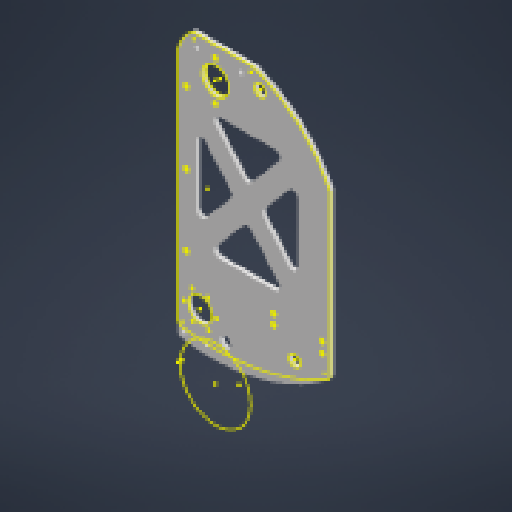
# Autodesk Inventor part: стенка пуляло ответная
Saved by Autodesk Inventor 2026.2 (Build 302298000, 298)
## iProperties
Created: 2025-11-22
Part Number: стенка пуляло ответная
Material: Типовые
Document SubType Name: Modeling
Designer: Phantom
Density: 1 g/cm^3
Appearance: По умолчанию
Author: Phantom
Autodesk Inventor part; units mm, degrees
ref_plane "YZ Plane" through (0, 0, 0) normal (1, 0, 0) x (0, 1, 0)
ref_plane "XZ Plane" through (0, 0, 0) normal (0, 1, 0) x (-1, 0, 0)
ref_plane "XY Plane" through (0, 0, 0) normal (0, 0, 1) x (1, 0, 0)
sketch "Эскиз1" plane through (0, 0, 0) normal (0, 0, 1) x (1, 0, 0)
  line L0 (0, 0) -> (150, 0)
  line L1 (150, 0) -> (150, 380)
  line L2 (150, 380) -> (0, 380)
  line L3 (0, 380) -> (0, 0)
  dimension "d2" = 150
  dimension "d3" = 380
  constraints: 8 end point, 2 parallel, 1 horizontal, 1 perpendicular
  measures "d2" distance of L1.end L2.end
  measures "d3" distance of L2.end L0.start
extrude "Выдавливание1" add sketch "Эскиз1" along normal blind 4
sketch "Эскиз3" plane through (0, 0, 0) normal (0, 0, -1) x (-1, 0, 0)
  circle A0 centre (-37, 259.345) radius 3.25
  line L0 (-150, 380) -> (0, 380) projected
  line L1 (0, 380) -> (0, 0) projected
  circle A1 centre (-37, 259.345) radius 203.5
  line L2 (-162.8639, 128.9118) -> (-165.6991, 126.0733) projected
  arc A2 (-165.6991, 126.0733) -> (-166.6166, 122.0185) centre (-139.5582, 118.0273) ccw projected
  arc A3 (-166.6166, 122.0185) -> (-165.4337, 121.2858) centre (-47.0897, 313.6766) ccw projected
  arc A4 (-165.4337, 121.2858) -> (-162.2121, 123.9136) centre (-181.0608, 143.7331) ccw projected
  arc A5 (-162.2121, 123.9136) -> (-161.041, 123.208) centre (-47.0897, 313.6766) ccw projected
  arc A6 (-161.041, 123.208) -> (-161.8583, 119.1318) centre (-134.7098, 115.8085) ccw projected
  arc A7 (-161.8583, 119.1318) -> (-160.6577, 118.4286) centre (-47.0897, 313.6766) ccw projected
  arc A8 (-160.6577, 118.4286) -> (-157.5019, 121.1349) centre (-176.8332, 140.484) ccw projected
  arc A9 (-157.5019, 121.1349) -> (-156.3138, 120.4584) centre (-47.0897, 313.6766) ccw projected
  arc A10 (-156.3138, 120.4584) -> (-157.0304, 116.3633) centre (-129.8082, 113.7098) ccw projected
  arc A11 (-157.0304, 116.3633) -> (-155.8129, 115.6898) centre (-47.0897, 313.6766) ccw projected
  arc A12 (-155.8129, 115.6898) -> (-152.7247, 118.473) centre (-172.5268, 137.34) ccw projected
  arc A13 (-152.7247, 118.473) -> (-151.5202, 117.826) centre (-47.0897, 313.6766) ccw projected
  arc A14 (-151.5202, 117.826) -> (-152.1357, 113.7145) centre (-124.8564, 111.7326) ccw projected
  arc A15 (-152.1357, 113.7145) -> (-150.902, 113.0712) centre (-47.0897, 313.6766) ccw projected
  arc A16 (-150.902, 113.0712) -> (-147.8833, 115.9297) centre (-168.1442, 134.3031) ccw projected
  arc A17 (-147.8833, 115.9297) -> (-146.6632, 115.3126) centre (-47.0897, 313.6766) ccw projected
  arc A18 (-146.6632, 115.3126) -> (-147.1773, 111.1871) centre (-119.8574, 109.8779) ccw projected
  arc A19 (-147.1773, 111.1871) -> (-145.928, 110.5745) centre (-47.0897, 313.6766) ccw projected
  arc A20 (-145.928, 110.5745) -> (-142.9807, 113.5064) centre (-163.6882, 131.375) ccw projected
  arc A21 (-142.9807, 113.5064) -> (-141.7458, 112.9195) centre (-47.0897, 313.6766) ccw projected
  arc A22 (-141.7458, 112.9195) -> (-142.1581, 108.7827) centre (-114.8143, 108.1469) ccw projected
  arc A23 (-142.1581, 108.7827) -> (-140.8941, 108.201) centre (-47.0897, 313.6766) ccw projected
  arc A24 (-140.8941, 108.201) -> (-138.0199, 111.2047) centre (-159.1613, 128.5577) ccw projected
  arc A25 (-138.0199, 111.2047) -> (-136.771, 110.6484) centre (-47.0897, 313.6766) ccw projected
  arc A26 (-136.771, 110.6484) -> (-137.0811, 106.5027) centre (-109.73, 106.5408) ccw projected
  arc A27 (-137.0811, 106.5027) -> (-135.8033, 105.9522) centre (-47.0897, 313.6766) ccw projected
  arc A28 (-135.8033, 105.9522) -> (-133.0039, 109.0259) centre (-154.5665, 125.8527) ccw projected
  arc A29 (-133.0039, 109.0259) -> (-131.7416, 108.5005) centre (-47.0897, 313.6766) ccw projected
  arc A30 (-131.7416, 108.5005) -> (-131.9496, 104.3484) centre (-104.6077, 105.0603) ccw projected
  arc A31 (-131.9496, 104.3484) -> (-130.6585, 103.8296) centre (-47.0897, 313.6766) ccw projected
  arc A32 (-130.6585, 103.8296) -> (-127.9358, 106.9713) centre (-149.9063, 123.2618) ccw projected
  arc A33 (-127.9358, 106.9713) -> (-126.6609, 106.4772) centre (-47.0897, 313.6766) ccw projected
  arc A34 (-126.6609, 106.4772) -> (-126.7665, 102.3212) centre (-99.4504, 103.7066) ccw projected
  arc A35 (-126.7665, 102.3212) -> (-125.4631, 101.8344) centre (-47.0897, 313.6766) ccw projected
  arc A36 (-125.4631, 101.8344) -> (-122.8185, 105.0422) centre (-145.1838, 120.7864) ccw projected
  arc A37 (-122.8185, 105.0422) -> (-121.5319, 104.5796) centre (-47.0897, 313.6766) ccw projected
  arc A38 (-121.5319, 104.5796) -> (-121.5351, 100.4223) centre (-94.2614, 102.4803) ccw projected
  arc A39 (-121.5351, 100.4223) -> (-120.22, 99.9678) centre (-47.0897, 313.6766) ccw projected
  arc A40 (-120.22, 99.9678) -> (-117.6553, 103.2397) centre (-140.4017, 118.4282) ccw projected
  arc A41 (-117.6553, 103.2397) -> (-116.3577, 102.8091) centre (-47.0897, 313.6766) ccw projected
  arc A42 (-116.3577, 102.8091) -> (-116.2584, 98.6529) centre (-89.0438, 101.3822) ccw projected
  arc A43 (-116.2584, 98.6529) -> (-114.9326, 98.2309) centre (-47.0897, 313.6766) ccw projected
  arc A44 (-114.9326, 98.2309) -> (-112.4493, 101.5651) centre (-135.5629, 116.1885) ccw projected
  arc A45 (-112.4493, 101.5651) -> (-111.1414, 101.1665) centre (-47.0897, 313.6766) ccw projected
  arc A46 (-111.1414, 101.1665) -> (-110.9398, 97.014) centre (-83.8006, 100.413) ccw projected
  arc A47 (-110.9398, 97.014) -> (-109.604, 96.6248) centre (-47.0897, 313.6766) ccw projected
  arc A48 (-109.604, 96.6248) -> (-107.2035, 100.0192) centre (-130.6705, 114.0687) ccw projected
  arc A49 (-107.2035, 100.0192) -> (-105.8863, 99.6529) centre (-47.0897, 313.6766) ccw projected
  arc A50 (-105.8863, 99.6529) -> (-105.5824, 95.5067) centre (-78.5352, 99.5733) ccw projected
  arc A51 (-105.5824, 95.5067) -> (-104.2374, 95.1505) centre (-47.0897, 313.6766) ccw projected
  arc A52 (-104.2374, 95.1505) -> (-101.9213, 98.603) centre (-125.7273, 112.0701) ccw projected
  arc A53 (-101.9213, 98.603) -> (-100.5954, 98.2693) centre (-47.0897, 313.6766) ccw projected
  arc A54 (-100.5954, 98.2693) -> (-100.1895, 94.1318) centre (-73.2507, 98.8635) ccw projected
  arc A55 (-100.1895, 94.1318) -> (-98.8361, 93.8089) centre (-47.0897, 313.6766) ccw projected
  arc A56 (-98.8361, 93.8089) -> (-96.6058, 97.3173) centre (-120.7363, 110.1938) ccw projected
  arc A57 (-96.6058, 97.3173) -> (-95.2721, 97.0164) centre (-47.0897, 313.6766) ccw projected
  arc A58 (-95.2721, 97.0164) -> (-94.7644, 92.8902) centre (-67.9503, 98.2842) ccw projected
  arc A59 (-94.7644, 92.8902) -> (-93.4034, 92.6007) centre (-47.0897, 313.6766) ccw projected
  arc A60 (-93.4034, 92.6007) -> (-91.2602, 96.1631) centre (-115.7007, 108.4411) ccw projected
  arc A61 (-91.2602, 96.1631) -> (-89.9195, 95.8951) centre (-47.0897, 313.6766) ccw projected
  arc A62 (-89.9195, 95.8951) -> (-89.3103, 91.7826) centre (-62.6373, 97.8356) ccw projected
  arc A63 (-89.3103, 91.7826) -> (-88.2236, 91.5786) centre (-47.0897, 313.6766) ccw projected
  line L3 (-88.2236, 91.5786) -> (-86.0083, 96.7219) projected
  line L4 (-86.0083, 96.7219) -> (-85.0766, 98.9705) projected
  arc A64 (-162.8639, 128.9118) -> (-85.0766, 98.9705) centre (-47.0897, 313.6766) ccw projected
  circle A65 centre (-47.0897, 313.6766) radius 225.875
  line L5 (-145.5079, 77.1409) -> (-145.5079, 75.5909) projected
  arc A66 (-145.5079, 75.5909) -> (-144.0079, 74.0909) centre (-144.0079, 75.5909) ccw projected
  line L6 (-144.0079, 74.0909) -> (-92.7079, 74.0909) projected
  arc A67 (-92.7079, 74.0909) -> (-91.2079, 75.5909) centre (-92.7079, 75.5909) ccw projected
  line L7 (-91.2079, 75.5909) -> (-91.2079, 77.1409) projected
  line L8 (-91.2079, 77.1409) -> (-93.3271, 77.1409) projected
  arc A68 (-93.3271, 81.1409) -> (-93.3271, 77.1409) centre (-94.3579, 79.1409) ccw projected
  line L9 (-93.3271, 81.1409) -> (-91.2079, 81.1409) projected
  line L10 (-91.2079, 81.1409) -> (-91.2079, 87.0409) projected
  line L11 (-91.2079, 87.0409) -> (-93.3271, 87.0409) projected
  arc A69 (-93.3271, 91.0409) -> (-93.3271, 87.0409) centre (-94.3579, 89.0409) ccw projected
  line L12 (-93.3271, 91.0409) -> (-91.2079, 91.0409) projected
  line L13 (-91.2079, 91.0409) -> (-91.2079, 92.5909) projected
  arc A70 (-91.2079, 92.5909) -> (-92.7079, 94.0909) centre (-92.7079, 92.5909) ccw projected
  line L14 (-92.7079, 94.0909) -> (-144.0079, 94.0909) projected
  arc A71 (-144.0079, 94.0909) -> (-145.5079, 92.5909) centre (-144.0079, 92.5909) ccw projected
  line L15 (-145.5079, 92.5909) -> (-145.5079, 91.0409) projected
  line L16 (-145.5079, 91.0409) -> (-143.3887, 91.0409) projected
  arc A72 (-143.3887, 87.0409) -> (-143.3887, 91.0409) centre (-142.3579, 89.0409) ccw projected
  line L17 (-143.3887, 87.0409) -> (-145.5079, 87.0409) projected
  line L18 (-145.5079, 87.0409) -> (-145.5079, 81.1409) projected
  line L19 (-145.5079, 81.1409) -> (-143.3887, 81.1409) projected
  arc A73 (-143.3887, 77.1409) -> (-143.3887, 81.1409) centre (-142.3579, 79.1409) ccw projected
  line L20 (-143.3887, 77.1409) -> (-145.5079, 77.1409) projected
  line L21 (-99.5079, 94.0709) -> (-137.8079, 94.0709) projected
  arc A74 (-98.5279, 93.0909) -> (-99.5079, 94.0709) centre (-99.5079, 93.0909) ccw projected
  line L22 (-98.5279, 75.0909) -> (-98.5279, 93.0909) projected
  arc A75 (-99.5079, 74.1109) -> (-98.5279, 75.0909) centre (-99.5079, 75.0909) ccw projected
  line L23 (-137.8079, 74.1109) -> (-99.5079, 74.1109) projected
  arc A76 (-138.7879, 75.0909) -> (-137.8079, 74.1109) centre (-137.8079, 75.0909) ccw projected
  line L24 (-138.7879, 93.0909) -> (-138.7879, 75.0909) projected
  arc A77 (-137.8079, 94.0709) -> (-138.7879, 93.0909) centre (-137.8079, 93.0909) ccw projected
  circle A78 centre (-142.3579, 79.1409) radius 2.25
  circle A79 centre (-142.3579, 89.0409) radius 2.25
  circle A80 centre (-94.3579, 79.1409) radius 2.25
  circle A81 centre (-94.3579, 89.0409) radius 2.25
  circle A82 centre (-37, 259.345) radius 13.25
  line L25 (-37, 259.345) -> (-37, 239.745)
  line L26 (-37, 239.745) -> (-37, 278.945)
  circle A83 centre (-37, 239.745) radius 2.1
  circle A84 centre (-37, 278.945) radius 2.1
  circle A85 centre (-22.0897, 66.1445) radius 19.3809
  line L27 (-22.0897, 66.1445) -> (-22.0897, 37.9965)
  circle A86 centre (-22.0897, 56.392) radius 12
  circle A87 centre (-13.8706, 70.1196) radius 1.6
  circle A88 centre (-6.0917, 56.1378) radius 1.6
  circle A89 centre (-14.3108, 42.4102) radius 1.6
  circle A90 centre (-30.3088, 42.6644) radius 1.6
  circle A91 centre (-38.0877, 56.6461) radius 1.6
  circle A92 centre (-29.8686, 70.3737) radius 1.6
  point P0 (-22.0897, 56.392)
  point P1 (-22.0897, 56.392)
  dimension "d7" = 407
  dimension "d4" = 6.5
  dimension "d5" = 120.655
  dimension "d6" = 37
  dimension "d10" = 26.5
  dimension "d11" = 19.6
  dimension "d12" = 39.2
  dimension "d13" = 4.2
  dimension "d14" = 4.2
  constraints: 16 centre point, 9 coincident, 6 end point, 4 concentric, 2 point on line, 2 vertical, 8 other
  measures "d4" diameter of A0
  measures "d5" distance from line of L0 A0.centre
  measures "d6" distance from line of L1 A0.centre
  measures "d10" diameter of A82
  measures "d11" distance of L25.start L25.end
  measures "d12" distance of L25.end L26.end
  measures "d13" diameter of A83
  measures "d14" diameter of A84
extrude "Выдавливание2" cut sketch "Эскиз3" against normal blind 10 contours A0 L25 L26 | L26 L25 A0 | A86 A85 L27 A1 | A1 A86 | A88 A85 | A85 A88 | L27 A85 A86 A1 | A91 A1 A85 | A85 A1 A91 | L27 A86 A85 | A85 A86 L27 | A91 A85 A1 | A85 A91 A1 | A81 A69 | A79 A72 | A73 A78 | A80 A68 | A87 | A89 | A90 | A92
sketch "Эскиз4" plane through (0, 0, 0) normal (0, 0, -1) x (-1, 0, 0)
  circle A0 centre (-37, 259.345) radius 13.25 projected
  circle A1 centre (-37, 278.945) radius 2.1 projected
  circle A2 centre (-37, 239.745) radius 2.1 projected
  point P0 (0, 0)
extrude "Выдавливание3" cut sketch "Эскиз3" against normal blind 10 contours A0 L25 L26 | A0 L26 A82 L25 | L26 L25 A0 | A0 L25 A82 L26 | A83 | A84
sketch "Эскиз5" plane through (150, 0, 0) normal (1, 0, 0) x (0, 0, -1)
  line L0 (-4, 380) -> (-4, 0) projected
  line L1 (-4, 30) -> (0, 30)
  line L2 (0, 0) -> (-4, 0) projected
  line L3 (-4, 290) -> (0, 290)
  line L4 (0, 0) -> (0, 380) projected
  line L5 (0, 380) -> (-4, 380) projected
  dimension "d17" = 30
  dimension "d18" = 90
  constraints: 4 end point, 3 point on line, 1 horizontal, 1 perpendicular
  measures "d17" distance between parallel lines of L2 L1
  measures "d18" distance between parallel lines of L3 L5
extrude "Выдавливание4" cut sketch "Эскиз5" against normal through all contours L5 L4 L3 L0 | L1 L4 L2 L0
sketch "Эскиз6" plane through (0, 0, 0) normal (0, 0, -1) x (-1, 0, 0)
  circle A0 centre (-37, 259.345) radius 13.25 projected
  circle A1 centre (-37, 259.345) radius 229.345
  line L0 (0, 30) -> (-150, 30) projected
  circle A2 centre (-37, 259.345) radius 37.9855
  line L1 (-150, 30) -> (-150, 290) projected
  arc A3 (-40.2154, 297.1942) -> (-150, 221.3595) centre (-28.8449, 163.3493) ccw
  circle A4 centre (-142.3579, 89.0409) radius 2.25 projected
  circle A5 centre (-94.3579, 79.1409) radius 2.25 projected
  circle A6 centre (-142.3579, 79.1409) radius 2.25 projected
  circle A7 centre (-94.3579, 89.0409) radius 2.25 projected
  circle A8 centre (-37, 259.345) radius 13.25 projected
  circle A9 centre (-37, 278.945) radius 2.1 projected
  circle A10 centre (-37, 239.745) radius 2.1 projected
  line L2 (0, 290) -> (-150, 290) projected
  line L3 (-150, 30) -> (-150, 290) projected
  line L4 (-150, 30) -> (0, 30) projected
  line L5 (0, 290) -> (0, 30) projected
  point P0 (0, 0)
  point P1 (0, 267.9415)
  point P2 (-14.5685, 290)
  point P3 (-73.6036, 290)
  point P4 (0, 33.0043)
  point P5 (-37, 30)
  point P6 (-150, 59.7701)
  constraints: 2 centre point, 2 coincident, 2 point on circle, 1 point on line, 1 tangent, 4 other
extrude "Выдавливание5" cut sketch "Эскиз6" against normal blind 10 contours A1 L0 L1 | L5 L0 A1 | L1 L2 A3 | A2 L2 L5 picked at (-4.9355, 285.277)
fillet "Сопряжение1" radius 5 4 edges at (73.6036, 290, 2) (14.5685, 290, 2) (150, 59.7701, 2) (0, 33.0043, 2)
sketch "Эскиз7" plane through (0, 0, 0) normal (0, 0, -1) x (-1, 0, 0)
  circle A0 centre (-37, 259.345) radius 35 projected
  circle A1 centre (-81, 273) radius 5.5
  line L0 (-16.2668, 290) -> (-72.7377, 290) projected
  circle A2 centre (-115, 59.0909) radius 5.5
  line L1 (-150, 62.7066) -> (-150, 221.3595) projected
  line L2 (-144.0079, 74.0909) -> (-92.7079, 74.0909) projected
  point P0 (0, 0)
  dimension "d24" = 11
  dimension "d25" = 17
  dimension "d26" = 44
  dimension "d27" = 11
  dimension "d28" = 35
  dimension "d29" = 15
  constraints: 2 centre point
  measures "d24" diameter of A1
  measures "d25" distance from line of A1.centre L0
  measures "d26" horizontal distance of A0.centre A1.centre
  measures "d27" diameter of A2
  measures "d28" distance from line of A2.centre L1
  measures "d29" distance from line of A2.centre L2
extrude "Выдавливание6" cut sketch "Эскиз7" against normal blind 10 contours A1 | A2
sketch "Эскиз8" plane through (0, 0, 0) normal (0, 0, -1) x (-1, 0, 0)
  line L0 (0, 167.3772) -> (0, 171.6772) projected
  line L1 (0, 169.5272) -> (-8, 169.5272)
  line L2 (0, 97.0611) -> (0, 101.3611) projected
  line L3 (0, 237.7901) -> (0, 242.0901) projected
  line L4 (0, 239.9401) -> (-8, 239.9401)
  line L5 (0, 99.2111) -> (-8, 99.2111)
  circle A0 centre (-8, 99.2111) radius 2.25
  circle A1 centre (-8, 169.5272) radius 2.25
  circle A2 centre (-8, 239.9401) radius 2.25
  point P0 (0, 0)
  dimension "d32" = 8
  dimension "d33" = 4.5
  dimension "d34" = 8
  dimension "d35" = 8
  constraints: 6 end point, 3 centre point, 3 coincident, 3 horizontal, 3 midpoint
  measures "d32" distance of L5.start L5.end
  measures "d33" diameter of A0
  measures "d34" distance of L1.start L1.end
  measures "d35" distance of L4.start L4.end
extrude "Выдавливание7" cut sketch "Эскиз8" against normal blind 10
sketch "Эскиз9" plane through (0, 0, 0) normal (0, 0, -1) x (-1, 0, 0)
  point P0 (0, 0)
sketch "Эскиз10" plane through (0, 0, 4) normal (0, 0, 1) x (1, 0, 0)
  arc A0 (60.9055, 10.4177) -> (61.5221, 11.6904) centre (60.5775, 11.3623) ccw projected
  circle A1 centre (8, 239.9401) radius 2.25 projected
  circle A2 centre (8, 169.5272) radius 2.25 projected
  circle A3 centre (8, 99.2111) radius 2.25 projected
  circle A4 centre (81, 273) radius 5.5 projected
  circle A5 centre (115, 59.0909) radius 5.5 projected
  arc A6 (0, 37.2939) -> (4.2868, 32.3451) centre (5, 37.2939) ccw projected
  arc A7 (4.2868, 32.3451) -> (147.407, 58.3241) centre (37, 259.345) ccw projected
  arc A8 (147.407, 58.3241) -> (150, 62.7066) centre (145, 62.7066) ccw projected
  line L0 (150, 62.7066) -> (150, 221.3595) projected
  arc A9 (150, 221.3595) -> (74.4347, 289.7032) centre (28.8449, 163.3493) ccw projected
  arc A10 (74.4347, 289.7032) -> (72.7377, 290) centre (72.7377, 285) ccw projected
  line L1 (72.7377, 290) -> (16.2668, 290) projected
  arc A11 (16.2668, 290) -> (13.124, 288.8888) centre (16.2668, 285) ccw projected
  arc A12 (13.124, 288.8888) -> (0, 267.9415) centre (37, 259.345) ccw projected
  line L2 (0, 267.9415) -> (0, 37.2939) projected
  circle A13 centre (22.0897, 56.392) radius 12 projected
  circle A14 centre (13.8706, 70.1196) radius 1.6 projected
  circle A15 centre (142.3579, 79.1409) radius 2.25 projected
  circle A16 centre (142.3579, 89.0409) radius 2.25 projected
  circle A17 centre (6.0917, 56.1378) radius 1.6 projected
  circle A18 centre (29.8686, 70.3737) radius 1.6 projected
  circle A19 centre (30.3088, 42.6644) radius 1.6 projected
  circle A20 centre (94.3579, 89.0409) radius 2.25 projected
  circle A21 centre (94.3579, 79.1409) radius 2.25 projected
  circle A22 centre (14.3108, 42.4102) radius 1.6 projected
  circle A23 centre (38.0877, 56.6461) radius 1.6 projected
  circle A24 centre (37, 259.345) radius 13.25 projected
  circle A25 centre (37, 278.945) radius 2.1 projected
  circle A26 centre (37, 239.745) radius 2.1 projected
  point P0 (0, 0)
sketch "Эскиз11" plane through (0, 0, 4) normal (0, 0, 1) x (1, 0, 0)
  circle A0 centre (37, 0) radius 35 projected
  point P0 (0, 0)
sketch "Эскиз12" plane through (0, 0, 4) normal (0, 0, 1) x (1, 0, 0)
  circle A0 centre (46.8597, 40.7124) radius 5.5 projected
  circle A1 centre (46.8597, 40.7124) radius 5.5
  circle A2 centre (62, 278.7903) radius 2.1 projected
  circle A3 centre (19, 278.7903) radius 2.1 projected
  point P0 (0, 0)
  dimension "d38" = 11
  constraints: 1 centre point, 1 coincident
  measures "d38" diameter of A1
extrude "Выдавливание8" cut sketch "Эскиз12" against normal blind 10
sketch "Эскиз13" plane through (0, 0, 4) normal (0, 0, 1) x (1, 0, 0)
  circle A0 centre (27.8653, 29.2915) radius 2.1 projected
  circle A1 centre (5.75, 29.2915) radius 2.1 projected
  circle A2 centre (62, 278.7903) radius 2.1 projected
  circle A3 centre (19, 278.7903) radius 2.1 projected
  circle A4 centre (46.8597, 40.7124) radius 5.5 projected
  circle A5 centre (8, 239.9401) radius 2.25 projected
  circle A6 centre (8, 169.5272) radius 2.25 projected
  circle A7 centre (8, 99.2111) radius 2.25 projected
  circle A8 centre (81, 273) radius 5.5 projected
  circle A9 centre (115, 59.0909) radius 5.5 projected
  arc A10 (0, 27.3695) -> (4.2138, 22.4317) centre (5, 27.3695) ccw projected
  arc A11 (4.2138, 22.4317) -> (18.1652, 20.7422) centre (33.7733, 208.0855) ccw projected
  arc A12 (18.1652, 20.7422) -> (25.7653, 20.2638) centre (37, 259.345) ccw projected
  arc A13 (25.7653, 20.2638) -> (147.1688, 58.1436) centre (33.7733, 208.0855) ccw projected
  arc A14 (147.5924, 58.4311) -> (147.1688, 58.1436) centre (150.1848, 54.1556) ccw projected
  arc A15 (147.5924, 58.4311) -> (150, 62.7066) centre (145, 62.7066) ccw projected
  line L0 (150, 62.7066) -> (150, 221.3595) projected
  arc A16 (150, 221.3595) -> (74.4347, 289.7032) centre (28.8449, 163.3493) ccw projected
  arc A17 (74.4347, 289.7032) -> (72.7377, 290) centre (72.7377, 285) ccw projected
  line L1 (72.7377, 290) -> (16.2668, 290) projected
  arc A18 (16.2668, 290) -> (13.124, 288.8888) centre (16.2668, 285) ccw projected
  arc A19 (13.124, 288.8888) -> (0, 267.9415) centre (37, 259.345) ccw projected
  line L2 (0, 267.9415) -> (0, 27.3695) projected
  circle A20 centre (142.3579, 89.0409) radius 2.25 projected
  circle A21 centre (79.3261, 72.7806) radius 1.6 projected
  circle A22 centre (63.7683, 44.8172) radius 1.6 projected
  circle A23 centre (79.7662, 45.0713) radius 1.6 projected
  circle A24 centre (94.3579, 79.1409) radius 2.25 projected
  circle A25 centre (142.3579, 79.1409) radius 2.25 projected
  circle A26 centre (71.5472, 58.7989) radius 12 projected
  circle A27 centre (63.3281, 72.5265) radius 1.6 projected
  circle A28 centre (55.5492, 58.5447) radius 1.6 projected
  circle A29 centre (87.5451, 59.053) radius 1.6 projected
  circle A30 centre (94.3579, 89.0409) radius 2.25 projected
  circle A31 centre (37, 259.345) radius 13.25 projected
  circle A32 centre (37, 278.945) radius 2.1 projected
  circle A33 centre (37, 239.745) radius 2.1 projected
  arc A34 (4.2868, 32.3451) -> (147.407, 58.3241) centre (37, 259.345) ccw projected
  circle A35 centre (46.8597, 40.7124) radius 5.5 projected
  circle A36 centre (62, 278.7903) radius 2.1 projected
  circle A37 centre (19, 278.7903) radius 2.1 projected
  circle A38 centre (8, 239.9401) radius 2.25 projected
  circle A39 centre (8, 169.5272) radius 2.25 projected
  circle A40 centre (8, 99.2111) radius 2.25 projected
  circle A41 centre (81, 273) radius 5.5 projected
  circle A42 centre (115, 59.0909) radius 5.5 projected
  arc A43 (0, 37.2939) -> (4.2868, 32.3451) centre (5, 37.2939) ccw projected
  arc A44 (4.2868, 32.3451) -> (147.407, 58.3241) centre (37, 259.345) ccw projected
  arc A45 (147.407, 58.3241) -> (150, 62.7066) centre (145, 62.7066) ccw projected
  line L3 (150, 62.7066) -> (150, 221.3595) projected
  arc A46 (150, 221.3595) -> (74.4347, 289.7032) centre (28.8449, 163.3493) ccw projected
  arc A47 (74.4347, 289.7032) -> (72.7377, 290) centre (72.7377, 285) ccw projected
  line L4 (72.7377, 290) -> (16.2668, 290) projected
  arc A48 (16.2668, 290) -> (13.124, 288.8888) centre (16.2668, 285) ccw projected
  arc A49 (13.124, 288.8888) -> (0, 267.9415) centre (37, 259.345) ccw projected
  line L5 (0, 267.9415) -> (0, 37.2939) projected
  circle A50 centre (22.0897, 56.392) radius 12 projected
  circle A51 centre (13.8706, 70.1196) radius 1.6 projected
  circle A52 centre (142.3579, 79.1409) radius 2.25 projected
  circle A53 centre (142.3579, 89.0409) radius 2.25 projected
  circle A54 centre (6.0917, 56.1378) radius 1.6 projected
  circle A55 centre (29.8686, 70.3737) radius 1.6 projected
  circle A56 centre (30.3088, 42.6644) radius 1.6 projected
  circle A57 centre (94.3579, 89.0409) radius 2.25 projected
  circle A58 centre (94.3579, 79.1409) radius 2.25 projected
  circle A59 centre (14.3108, 42.4102) radius 1.6 projected
  circle A60 centre (38.0877, 56.6461) radius 1.6 projected
  circle A61 centre (37, 259.345) radius 13.25 projected
  circle A62 centre (37, 278.945) radius 2.1 projected
  circle A63 centre (37, 239.745) radius 2.1 projected
  line L6 (52.0917, 166.3314) -> (26.8046, 136.6761) projected
  arc A64 (18, 139.9204) -> (26.8046, 136.6761) centre (23, 139.9204) ccw projected
  line L7 (18, 139.9204) -> (18, 199.2309) projected
  arc A65 (26.8046, 202.4751) -> (18, 199.2309) centre (23, 199.2309) ccw projected
  line L8 (26.8046, 202.4751) -> (52.0917, 172.8198) projected
  arc A66 (52.0917, 166.3314) -> (52.0917, 172.8198) centre (48.2871, 169.5756) ccw projected
  line L9 (83.9083, 172.8198) -> (109.1954, 202.4751) projected
  arc A67 (118, 199.2309) -> (109.1954, 202.4751) centre (113, 199.2309) ccw projected
  line L10 (118, 199.2309) -> (118, 139.9204) projected
  arc A68 (109.1954, 136.6761) -> (118, 139.9204) centre (113, 139.9204) ccw projected
  line L11 (109.1954, 136.6761) -> (83.9083, 166.3314) projected
  arc A69 (83.9083, 172.8198) -> (83.9083, 166.3314) centre (87.7129, 169.5756) ccw projected
  line L12 (64.1954, 189.4495) -> (36.6988, 221.6959) projected
  arc A70 (40.5034, 229.9401) -> (36.6988, 221.6959) centre (40.5034, 224.9401) ccw projected
  line L13 (40.5034, 229.9401) -> (95.4966, 229.9401) projected
  arc A71 (99.3012, 221.6959) -> (95.4966, 229.9401) centre (95.4966, 224.9401) ccw projected
  line L14 (99.3012, 221.6959) -> (71.8046, 189.4495) projected
  arc A72 (64.1954, 189.4495) -> (71.8046, 189.4495) centre (68, 192.6937) ccw projected
  line L15 (71.8046, 149.7017) -> (99.3012, 117.4553) projected
  arc A73 (95.4966, 109.2111) -> (99.3012, 117.4553) centre (95.4966, 114.2111) ccw projected
  line L16 (95.4966, 109.2111) -> (40.5034, 109.2111) projected
  arc A74 (36.6988, 117.4553) -> (40.5034, 109.2111) centre (40.5034, 114.2111) ccw projected
  line L17 (36.6988, 117.4553) -> (64.1954, 149.7017) projected
  arc A75 (71.8046, 149.7017) -> (64.1954, 149.7017) centre (68, 146.4575) ccw projected
  point P0 (0, 0)
  point P1 (147.5924, 58.4311)
  point P2 (147.407, 58.3241)
  point P3 (29.7979, 30.1131)
  point P4 (26.0039, 30.2638)
  point P5 (4.2868, 32.3451)
  point P6 (0, 37.2939)
extrude "Выдавливание9" add sketch "Эскиз13" against normal up to surface (4 mm away) contours A0 A34 A45 A14 A13 A12 A11 A10 L2 A43
sketch "Эскиз14" plane through (0, 0, 4) normal (0, 0, 1) x (1, 0, 0)
  arc A0 (26.0039, 30.2638) -> (29.7979, 30.1131) centre (27.8653, 29.2915) ccw projected
  circle A1 centre (27.8653, 29.2915) radius 2.1
  point P0 (0, 0)
  constraints: 1 centre point, 1 coincident, 1 concentric
extrude "Выдавливание10" cut sketch "Эскиз14" against normal blind 10
sketch "Эскиз15" plane through (0, 0, 4) normal (0, 0, 1) x (1, 0, 0)
  point P0 (0, 0)
sketch "Эскиз16" plane through (0, 0, 4) normal (0, 0, 1) x (1, 0, 0)
  line L0 (52.0917, 166.3314) -> (26.8046, 136.6761) projected
  arc A0 (18, 139.9204) -> (26.8046, 136.6761) centre (23, 139.9204) ccw projected
  line L1 (18, 139.9204) -> (18, 199.2309) projected
  arc A1 (26.8046, 202.4751) -> (18, 199.2309) centre (23, 199.2309) ccw projected
  line L2 (26.8046, 202.4751) -> (52.0917, 172.8198) projected
  arc A2 (52.0917, 166.3314) -> (52.0917, 172.8198) centre (48.2871, 169.5756) ccw projected
  line L3 (83.9083, 172.8198) -> (109.1954, 202.4751) projected
  arc A3 (118, 199.2309) -> (109.1954, 202.4751) centre (113, 199.2309) ccw projected
  line L4 (118, 199.2309) -> (118, 139.9204) projected
  arc A4 (109.1954, 136.6761) -> (118, 139.9204) centre (113, 139.9204) ccw projected
  line L5 (109.1954, 136.6761) -> (83.9083, 166.3314) projected
  arc A5 (83.9083, 172.8198) -> (83.9083, 166.3314) centre (87.7129, 169.5756) ccw projected
  line L6 (64.1954, 189.4495) -> (36.6988, 221.6959) projected
  arc A6 (40.5034, 229.9401) -> (36.6988, 221.6959) centre (40.5034, 224.9401) ccw projected
  line L7 (40.5034, 229.9401) -> (95.4966, 229.9401) projected
  arc A7 (99.3012, 221.6959) -> (95.4966, 229.9401) centre (95.4966, 224.9401) ccw projected
  line L8 (99.3012, 221.6959) -> (71.8046, 189.4495) projected
  arc A8 (64.1954, 189.4495) -> (71.8046, 189.4495) centre (68, 192.6937) ccw projected
  line L9 (71.8046, 149.7017) -> (99.3012, 117.4553) projected
  arc A9 (95.4966, 109.2111) -> (99.3012, 117.4553) centre (95.4966, 114.2111) ccw projected
  line L10 (95.4966, 109.2111) -> (40.5034, 109.2111) projected
  arc A10 (36.6988, 117.4553) -> (40.5034, 109.2111) centre (40.5034, 114.2111) ccw projected
  line L11 (36.6988, 117.4553) -> (64.1954, 149.7017) projected
  arc A11 (71.8046, 149.7017) -> (64.1954, 149.7017) centre (68, 146.4575) ccw projected
  circle A12 centre (27.8653, 29.2915) radius 2.1 projected
  circle A13 centre (5.75, 29.2915) radius 2.1 projected
  circle A14 centre (62, 278.7903) radius 2.1 projected
  circle A15 centre (19, 278.7903) radius 2.1 projected
  circle A16 centre (46.8597, 40.7124) radius 5.5 projected
  circle A17 centre (8, 239.9401) radius 2.25 projected
  circle A18 centre (8, 169.5272) radius 2.25 projected
  circle A19 centre (8, 99.2111) radius 2.25 projected
  circle A20 centre (81, 273) radius 5.5 projected
  circle A21 centre (115, 59.0909) radius 5.5 projected
  arc A22 (0, 27.3695) -> (4.2138, 22.4317) centre (5, 27.3695) ccw projected
  arc A23 (4.2138, 22.4317) -> (18.1652, 20.7422) centre (33.7733, 208.0855) ccw projected
  arc A24 (18.1652, 20.7422) -> (25.7653, 20.2638) centre (37, 259.345) ccw projected
  arc A25 (25.7653, 20.2638) -> (147.1688, 58.1436) centre (33.7733, 208.0855) ccw projected
  arc A26 (147.5924, 58.4311) -> (147.1688, 58.1436) centre (150.1848, 54.1556) ccw projected
  arc A27 (147.5924, 58.4311) -> (150, 62.7066) centre (145, 62.7066) ccw projected
  line L12 (150, 62.7066) -> (150, 221.3595) projected
  arc A28 (150, 221.3595) -> (74.4347, 289.7032) centre (28.8449, 163.3493) ccw projected
  arc A29 (74.4347, 289.7032) -> (72.7377, 290) centre (72.7377, 285) ccw projected
  line L13 (72.7377, 290) -> (16.2668, 290) projected
  arc A30 (16.2668, 290) -> (13.124, 288.8888) centre (16.2668, 285) ccw projected
  arc A31 (13.124, 288.8888) -> (0, 267.9415) centre (37, 259.345) ccw projected
  line L14 (0, 267.9415) -> (0, 27.3695) projected
  circle A32 centre (142.3579, 89.0409) radius 2.25 projected
  circle A33 centre (79.3261, 72.7806) radius 1.6 projected
  circle A34 centre (63.7683, 44.8172) radius 1.6 projected
  circle A35 centre (79.7662, 45.0713) radius 1.6 projected
  circle A36 centre (94.3579, 79.1409) radius 2.25 projected
  circle A37 centre (142.3579, 79.1409) radius 2.25 projected
  circle A38 centre (71.5472, 58.7989) radius 12 projected
  circle A39 centre (63.3281, 72.5265) radius 1.6 projected
  circle A40 centre (55.5492, 58.5447) radius 1.6 projected
  circle A41 centre (87.5451, 59.053) radius 1.6 projected
  circle A42 centre (94.3579, 89.0409) radius 2.25 projected
  circle A43 centre (37, 259.345) radius 13.25 projected
  circle A44 centre (37, 278.945) radius 2.1 projected
  circle A45 centre (37, 239.745) radius 2.1 projected
  point P0 (0, 0)
extrude "Выдавливание11" cut sketch "Эскиз16" against normal blind 10 contours L0 A0 L1 A1 L2 A2 | L3 A3 L4 A4 L5 A5 | L6 A6 L7 A7 L8 A8 | L9 A9 L10 A10 L11 A11
